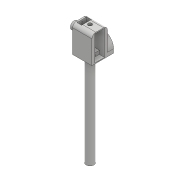
# Autodesk Inventor part: core_structure
Saved by Autodesk Inventor 2018 (Build 220112000, 112)
## iProperties
Created: 2018-02-12
Part Number: core_structure
Material: Generic
Document SubType Name: Modeling
Designer: Bardo91
Density: 1 g/cm^3
Appearance: Default
Author: Bardo91
Autodesk Inventor part; units mm, degrees
ref_plane "YZ Plane" through (0, 0, 0) normal (1, 0, 0) x (0, 1, 0)
ref_plane "XZ Plane" through (0, 0, 0) normal (0, 1, 0) x (-1, 0, 0)
ref_plane "XY Plane" through (0, 0, 0) normal (0, 0, 1) x (1, 0, 0)
sketch "Sketch1" plane through (0, 0, 0) normal (0, 0, 1) x (1, 0, 0)
  line L0 (0, 0) -> (25, 0)
  line L1 (25, 0) -> (25, 20)
  line L2 (25, 20) -> (0, 20)
  line L3 (0, 20) -> (0, 0)
  dimension "d0" = 25
  dimension "d1" = 20
  constraints: 8 end point, 2 perpendicular, 1 horizontal, 1 vertical
  measures "d0" distance of L0.start L0.end
  measures "d1" distance of L0.end L1.end
extrude "base" add sketch "Sketch1" along normal blind 35
sketch "Sketch4" plane through (0, 0, 0) normal (0, 0, -1) x (-1, 0, 0)
  line L0 (-25, 20) -> (0, 20) projected
  line L1 (-12.5, 20) -> (-12.5, 10)
  circle A0 centre (-12.5, 10) radius 5
  line L2 (-25, 0) -> (-25, 20) projected
  line L3 (-25, 20) -> (-25, 0)
  point P0 (0, 0)
  point P1 (-13, 32)
  point P2 (-5, 32)
  point P3 (0, 20)
  dimension "d18" = 10
  dimension "d19" = 10
  dimension "d92" = 20
  constraints: 4 end point, 1 centre point, 1 coincident, 1 collinear, 1 vertical, 2 other
  measures "d18" distance of L1.start L1.end
  measures "d19" diameter of A0
  measures "d92" distance of L2.start L2.end
extrude "attacher" add sketch "Sketch4" along normal blind 120
fillet "Fillet2" radius 4 1 edges at (17.5, 10, 0)
sketch "Sketch5" plane through (12.5, 10, -120) normal (0, 0, -1) x (-1, 0, 0)
  circle A0 centre (0, 0) radius 2.5
  point P0 (12.5, -10)
  dimension "d23" = 5
  constraints: 1 centre point
  measures "d23" diameter of A0
extrude "hole_bar_rigify" cut sketch "Sketch5" against normal through all
sketch "Sketch15" plane through (25, 0, 0) normal (1, 0, 0) x (0, 0, -1)
  line L0 (-35, 0) -> (-35, 20) projected
  line L1 (-35, 10) -> (0, 10)
  line L2 (-17.5, 10) -> (-17.5, 16.25)
  line L3 (-17.5, 16.25) -> (-29.1, 16.25)
  line L4 (-29.1, 16.25) -> (-29.1, 3.75)
  line L5 (-29.1, 3.75) -> (-5.9, 3.75)
  line L6 (-5.9, 3.75) -> (-5.9, 16.25)
  line L7 (-5.9, 16.25) -> (-17.5, 16.25)
  point P0 (0, 0)
  dimension "d76" = 6.25
  dimension "d77" = 11.6
  dimension "d78" = 12.5
  dimension "d79" = 23.2
  constraints: 14 end point, 5 perpendicular, 2 midpoint, 1 horizontal, 1 point on line, 1 vertical
  measures "d76" distance of L2.start L2.end
  measures "d77" distance of L2.end L3.end
  measures "d78" distance of L3.end L4.end
  measures "d79" distance of L4.end L5.end
extrude "servo_place" cut sketch "Sketch15" against normal blind 23
sketch "Sketch16" plane through (25, 0, 0) normal (1, 0, 0) x (0, 0, -1)
  line L0 (-5.9, 3.75) -> (-29.1, 3.75) projected
  line L1 (-29.1, 3.75) -> (-33.8, 3.75)
  line L2 (-33.8, 3.75) -> (-33.8, 16.25)
  line L3 (-29.1, 16.25) -> (-5.9, 16.25) projected
  line L4 (-33.8, 16.25) -> (-29.1, 16.25)
  line L5 (-29.1, 16.25) -> (-29.1, 3.75)
  line L6 (-5.9, 16.25) -> (-5.9, 3.75) projected
  line L7 (-5.9, 3.75) -> (-5.9, 16.25)
  line L8 (-5.9, 16.25) -> (-1.2, 16.25)
  line L9 (-1.2, 16.25) -> (-1.2, 3.75)
  line L10 (-1.2, 3.75) -> (-5.9, 3.75)
  point P0 (0, 0)
  dimension "d82" = 4.7
  dimension "d83" = 4.7
  constraints: 16 end point, 7 perpendicular, 1 horizontal
  measures "d82" distance of L0.end L1.end
  measures "d83" distance of L3.end L8.end
extrude "servo_place_2" cut sketch "Sketch16" against normal blind 6.6 contours L6 L8 L9 L10 | L1 L2 L4 L5
sketch "Sketch17" plane through (18.4, 0, 0) normal (1, 0, 0) x (0, 0, -1)
  line L0 (-33.8, 3.75) -> (-33.8, 16.25) projected
  line L1 (-33.8, 10) -> (-31.9, 10)
  line L2 (-1.2, 16.25) -> (-1.2, 3.75) projected
  line L3 (-1.2, 10) -> (-3.1, 10)
  circle A0 centre (-3.1, 10) radius 1
  circle A1 centre (-31.9, 10) radius 1
  point P0 (0, 0)
  dimension "d86" = 1.9
  dimension "d87" = 1.9
  dimension "d88" = 2
  dimension "d89" = 2
  constraints: 4 end point, 2 centre point, 2 coincident, 2 horizontal, 2 midpoint
  measures "d86" distance of L1.start L1.end
  measures "d87" distance of L3.start L3.end
  measures "d88" diameter of A0
  measures "d89" diameter of A1
extrude "screw_holes" cut sketch "Sketch17" against normal through all
fillet "Fillet3" radius 5 2 edges at (12.5, 20, 35) (12.5, 0, 35)
sketch "Sketch18" plane through (0, 0, 0) normal (-1, 0, 0) x (0, 0, 1)
  line L0 (35, 12.5) -> (35, 7.5) projected
  line L1 (35, 10) -> (24, 10)
  circle A0 centre (24, 10) radius 5
  point P0 (0, 0)
  dimension "d94" = 11
  dimension "d95" = 10
  constraints: 2 end point, 1 centre point, 1 coincident, 1 horizontal, 1 midpoint
  measures "d94" distance of L1.start L1.end
  measures "d95" diameter of A0
extrude "rot_axis" add sketch "Sketch18" along normal blind 8
sketch "Sketch20" plane through (-8, 10, 24) normal (-1, 0, 0) x (0, 0, 1)
  circle A0 centre (0, 0) radius 2.5
  point P0 (-24, -10)
  dimension "d102" = 5
  constraints: 1 centre point
  measures "d102" diameter of A0
extrude "rot_axis_hole" cut sketch "Sketch20" against normal up to surface (10 mm away)
sketch "Sketch21" plane through (2, 3.75, 29.1) normal (0, 0, -1) x (-1, 0, 0)
  line L0 (-16.4, 12.5) -> (0, 12.5) projected
  line L1 (0, 12.5) -> (-6, 12.5)
  line L2 (-6, 12.5) -> (-6, 0)
  line L3 (-16.4, 0) -> (0, 0) projected
  line L4 (-6, 0) -> (0, 0)
  line L5 (0, 12.5) -> (0, 0) projected
  line L6 (0, 0) -> (0, 12.5)
  point P0 (2, -3.75)
  dimension "d105" = 6
  constraints: 8 end point, 2 perpendicular, 2 point on line, 1 collinear
  measures "d105" distance of L0.end L1.end
extrude "cable_hole" cut sketch "Sketch21" against normal through all
fillet "Fillet5" radius 6 1 edges at (8, 10, 29.1)
sketch "Sketch22" plane through (0, 20, 0) normal (0, 1, 0) x (1, 0, 0)
  line L0 (0, 0) -> (0, -30) projected
  line L1 (0, -30) -> (0, -20)
  line L2 (0, -20) -> (0, -15)
  line L3 (0, -15) -> (5, -15)
  line L4 (5, -15) -> (5, -20)
  line L5 (5, -20) -> (10, -20)
  line L6 (10, -20) -> (10, -5)
  line L7 (10, -5) -> (5, -5)
  line L8 (5, -5) -> (5, -15)
  line L9 (10, -5) -> (25, -5)
  line L10 (25, -5) -> (25, 0)
  line L11 (25, 0) -> (10, 0)
  line L12 (10, 0) -> (10, -5)
  dimension "d109" = 10
  dimension "d110" = 5
  dimension "d111" = 5
  dimension "d112" = 5
  dimension "d113" = 5
  dimension "d114" = 15
  dimension "d115" = 15
  dimension "d116" = 5
  dimension "d117" = 15
  constraints: 24 end point, 6 perpendicular, 2 horizontal, 2 point on line, 1 midpoint
  measures "d109" distance of L0.end L1.end
  measures "d110" distance of L1.end L2.end
  measures "d111" distance of L2.end L3.end
  measures "d112" distance of L3.end L4.end
  measures "d113" distance of L4.end L5.end
  measures "d114" distance of L5.end L6.end
  measures "d115" distance of L6.end L9.end
  measures "d116" distance of L9.end L10.end
  measures "d117" distance of L10.end L11.end
extrude "cable_guide_1" add sketch "Sketch22" along normal blind 8
sketch "Sketch23" plane through (10, 20, 20) normal (1, 0, 0) x (0, 0, -1)
  line L0 (15, 0) -> (0, 0) projected
  line L1 (0, 0) -> (2, 0)
  line L2 (2, 0) -> (13, 0)
  line L3 (13, 0) -> (13, 7)
  line L4 (13, 7) -> (2, 7)
  line L5 (2, 7) -> (2, 0)
  point P0 (20, -20)
  dimension "d120" = 2
  dimension "d121" = 11
  dimension "d122" = 7
  constraints: 10 end point, 3 perpendicular, 2 point on line
  measures "d120" distance of L0.end L1.end
  measures "d121" distance of L1.end L2.end
  measures "d122" distance of L2.end L3.end
sketch "Sketch24" plane through (10, 20, 5) normal (0, 0, 1) x (1, 0, 0)
  line L0 (0, 0) -> (2, 0)
  line L1 (15, 0) -> (0, 0) projected
  line L2 (2, 0) -> (13, 0)
  line L3 (13, 0) -> (13, 7)
  line L4 (13, 7) -> (2, 7)
  line L5 (2, 7) -> (2, 0)
  point P0 (-10, -20)
  dimension "d123" = 2
  dimension "d124" = 11
  dimension "d125" = 7
  constraints: 10 end point, 2 perpendicular, 2 point on line, 1 vertical
  measures "d123" distance of L0.start L0.end
  measures "d124" distance of L0.end L2.end
  measures "d125" distance of L2.end L3.end
extrude "cable_guide_2" cut sketch "Sketch23" against normal blind 8
extrude "cable_guide_3" cut sketch "Sketch24" against normal blind 8
sketch "Sketch25" plane through (10, 20, 5) normal (1, 0, 0) x (0, 0, -1)
  line L0 (5, 8) -> (0, 8) projected
  line L1 (0, 0) -> (0, 8) projected
  line L2 (0, 8) -> (0, 0)
  line L3 (-2, 0) -> (-2, 7) projected
  line L4 (0, 0) -> (-2, 0)
  line L5 (-2, 0) -> (-2, 7)
  line L6 (-13, 7) -> (-2, 7) projected
  line L7 (-2, 7) -> (-13, 7)
  line L8 (-13, 7) -> (-13, 0)
  line L9 (-15, 0) -> (-13, 0) projected
  line L10 (-13, 0) -> (-15, 0)
  line L11 (-15, 0) -> (-15, 8)
  line L12 (-15, 8) -> (0, 8)
  point P0 (5, -20)
  constraints: 16 end point, 7 perpendicular, 1 collinear, 1 point on line
revolve "cable_guide_4" add sketch "Sketch25" angle 90 about axis through (10, 20, 5) along (0, 1, 0)
equation "\"d18\" = 0.5 * d92"
body "Solid1"
